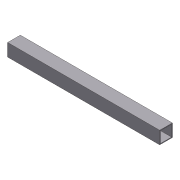
# Autodesk Inventor part: Frame_UpperFrameSupport_Rear
Saved by Autodesk Inventor 2012 (Build 160160000, 160)
## iProperties
Created: 2012-01-18
Part Number: Frame_UpperFrameSupport_Rear
Material: Aluminum-6061
Document SubType Name: Modeling
Designer: JesseK
Mass: 124.9 g
Surface Area: 583.668 cm^2
Volume: 46.0886 cm^3
Density: 2.71 g/cm^3
Author: JesseK
Autodesk Inventor part; units mm, degrees
ref_plane "YZ Plane" through (0, 0, 0) normal (1, 0, 0) x (0, 1, 0)
ref_plane "XZ Plane" through (0, 0, 0) normal (0, 1, 0) x (-1, 0, 0)
ref_plane "XY Plane" through (0, 0, 0) normal (0, 0, 1) x (1, 0, 0)
sketch "Sketch1" plane through (0, 0, 0) normal (0, 0, 1) x (1, 0, 0)
  line L0 (0, 0) -> (0, 25.4)
  line L1 (0, 25.4) -> (304.8, 25.4)
  line L2 (304.8, 25.4) -> (304.8, 0)
  line L3 (304.8, 0) -> (0, 0)
  dimension "d5" = 25.4
  dimension "d6" = 304.8
  constraints: 8 end point, 2 vertical, 1 horizontal, 1 parallel
  measures "d5" distance between parallel lines of L3 L1
  measures "d6" distance between parallel lines of L0 L2
extrude "Extrusion1" add sketch "Sketch1" along normal blind 25.4
shell "Shell2" thickness 1.5875 removed faces 2 at (0, 8.4667, 8.4667) at (304.8, 16.9333, 8.4667)
body "Solid1"
